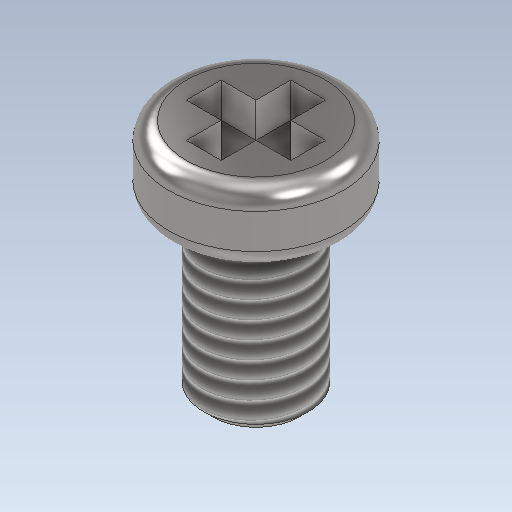
# Autodesk Inventor part: M3_Smaller_Bolt
Saved by Autodesk Inventor 2021 (Build 250183000, 183)
## iProperties
Created: 2020-03-26
Part Number: M3_Smaller_Bolt
Material: Steel, Alloy
Document SubType Name: Modeling
Designer: ermoz
Density: 7.73 g/cm^3
Appearance: Semi-Polished
Mass: 0.50985 g
Surface Area: 1.19028 cm^2
Volume: 0.0659573 cm^3
Author: ermoz
Autodesk Inventor part; units mm, degrees
ref_plane "YZ Plane" through (0, 0, 0) normal (1, 0, 0) x (0, 1, 0)
ref_plane "XZ Plane" through (0, 0, 0) normal (0, 1, 0) x (-1, 0, 0)
ref_plane "XY Plane" through (0, 0, 0) normal (0, 0, 1) x (1, 0, 0)
sketch "Sketch1" plane through (0, 0, 0) normal (0, 1, 0) x (-1, 0, 0)
  circle A0 centre (0, 0) radius 1.5
  dimension "d0" = 3
  constraints: 1 centre point, 1 coincident
  measures "d0" diameter of A0
extrude "Extrusion1" add sketch "Sketch1" along normal blind 4.75
sketch "Sketch2" plane through (0, 4.75, 0) normal (0, 1, 0) x (1, 0, 0)
  circle A0 centre (0, 0) radius 2.5
  dimension "d3" = 5
  constraints: 1 centre point, 1 coincident
  measures "d3" diameter of A0
extrude "Extrusion2" add sketch "Sketch2" along normal blind 2
fillet "Fillet1" radius 0.5 2 edges at (-2.5, 6.75, 0) (-2.5, 4.75, 0)
sketch "Sketch3" plane through (0, 6.75, 0) normal (0, 1, 0) x (1, 0, 0)
  line L0 (0.5, -1.5) -> (-0.5, -1.5)
  line L1 (-0.5, -1.5) -> (-0.5, 1.5)
  line L2 (-0.5, 1.5) -> (0.5, 1.5)
  line L3 (0.5, 1.5) -> (0.5, -1.5)
  line L4 (0.5, -1.5) -> (-0.5, 1.5) construction
  line L5 (-0.5, -1.5) -> (0.5, 1.5) construction
  line L6 (-1.5, -0.5) -> (1.5, -0.5)
  line L7 (1.5, -0.5) -> (1.5, 0.5)
  line L8 (1.5, 0.5) -> (-1.5, 0.5)
  line L9 (-1.5, 0.5) -> (-1.5, -0.5)
  line L10 (-1.5, -0.5) -> (1.5, 0.5) construction
  line L11 (1.5, -0.5) -> (-1.5, 0.5) construction
  point P0 (0, 0)
  point P1 (-0.5, -0.5)
  point P2 (0.5, -0.5)
  point P3 (0.5, 0.5)
  point P4 (-0.5, 0.5)
  dimension "d7" = 1
  dimension "d8" = 3
  dimension "d9" = 3
  dimension "d10" = 1
  constraints: 24 end point, 4 midpoint, 4 parallel, 2 horizontal, 2 perpendicular
  measures "d7" distance of L1.end L2.end
  measures "d8" distance of L0.end L1.end
  measures "d9" distance of L8.end L7.end
  measures "d10" distance of L7.end L6.end
extrude "Extrusion3" cut sketch "Sketch3" against normal blind 1
thread "Thread1" size "M3x0.5" class "6g" standard "ANSI Metric M Profile" full length
chamfer "Chamfer1" distance 0.25 angle 45 1 edges at (1.5, 0, 0)
body "Solid1"
